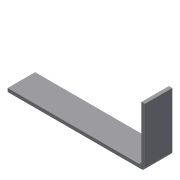
# Autodesk Inventor part: rollerbracketer
Saved by Autodesk Inventor 2015 (Build 190159000, 159)
## iProperties
Created: 2015-03-13
Part Number: rollerbracketer
Material: Generic
Document SubType Name: Modeling
Designer: Jaden
Density: 1 g/cm^3
Appearance: Default
Author: Jaden
Autodesk Inventor part; units mm, degrees
ref_plane "YZ Plane" through (0, 0, 0) normal (1, 0, 0) x (0, 1, 0)
ref_plane "XZ Plane" through (0, 0, 0) normal (0, 1, 0) x (-1, 0, 0)
ref_plane "XY Plane" through (0, 0, 0) normal (0, 0, 1) x (1, 0, 0)
sketch "Sketch1" plane through (0, 0, 0) normal (0, 0, 1) x (1, 0, 0)
  line L0 (0, 0) -> (104.775, 0)
  line L1 (0, 3.175) -> (101.6, 3.175)
  line L2 (104.775, 6.35) -> (104.775, 53.975)
  line L3 (104.775, 53.975) -> (107.95, 53.975)
  line L4 (107.95, 53.975) -> (107.95, 3.175)
  line L5 (104.775, 0) -> (104.775, 0)
  arc A0 (101.6, 3.175) -> (104.775, 6.35) centre (101.6, 6.35) ccw
  arc A1 (104.775, 0) -> (107.95, 3.175) centre (104.775, 3.175) ccw
  line L6 (0, 3.175) -> (-19.05, 3.175)
  line L7 (-19.05, 3.175) -> (-19.05, 0)
  line L8 (-19.05, 0) -> (0, 0)
  point P0 (104.775, 3.175)
  dimension "d0" = 3.175
  dimension "d2" = 50.8
  dimension "d3" = 90
  dimension "d4" = 3.175
  dimension "d5" = 3.175
  dimension "d8" = 19.05
  constraints: 18 end point, 5 perpendicular, 4 point on circle, 4 tangent, 3 horizontal, 2 centre point, 2 point on line, 1 collinear, 1 equal radius
  measures "d0" distance of L0.start L1.start
  measures "d2" distance of point (104.775, 3.175) L2.end
  measures "d3" angle of L2 L1
  measures "d4" distance of L2.end L3.end
  measures "d5" radius of A0
  measures "d8" distance of L1.start L6.end
extrude "Extrusion2" add sketch "Sketch1" along normal blind 25.4
body "Solid2"
